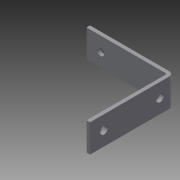
# Autodesk Inventor part: Gusset
Saved by Autodesk Inventor 2013 (Build 170138000, 138)
## iProperties
Created: 2013-01-31
Part Number: Gusset
Material: Generic
Document SubType Name: Sheet Metal
Designer: actoennies
Density: 1 g/cm^3
Flat Pattern Width: 2.54 cm
Flat Pattern Length: 14.7699 cm
Flat Pattern Area: 37.5156 cm^2
Sheet Metal Rule: Default
Sheet Metal Width: 1.000 in
Sheet Metal Length: 5.815 in
Sheet Metal Area: 5.815 in^2
Mass: 11.48 g
Surface Area: 86.0215 cm^2
Volume: 11.48 cm^3
Author: actoennies
Autodesk Inventor part; units mm, degrees
note: some values were not read from the file. Left out: dimensions or parameters whose unit could not be read.
ref_plane "YZ Plane" through (0, 0, 0) normal (1, 0, 0) x (0, 1, 0)
ref_plane "XZ Plane" through (0, 0, 0) normal (0, 1, 0) x (-1, 0, 0)
ref_plane "XY Plane" through (0, 0, 0) normal (0, 0, 1) x (1, 0, 0)
sketch "Sketch1" plane through (0, 0, 0) normal (0, 0, 1) x (1, 0, 0)
  line L0 (0, 0) -> (147.699314, 0)
  line L1 (147.699314, -25.4) -> (0, -25.4)
  line L2 (0, 0) -> (73.8378, 0)
  line L3 (73.8378, 0) -> (73.8378, -3.175)
  line L4 (73.8378, -3.175) -> (72.2503, -3.175)
  line L5 (72.2503, -3.175) -> (72.2503, -9.525)
  line L6 (72.2503, -9.525) -> (75.4253, -9.525)
  line L7 (75.4253, -9.525) -> (75.4253, -3.175)
  line L8 (75.4253, -3.175) -> (73.8378, -3.175)
  line L9 (73.849657, -25.4) -> (73.849657, -22.225)
  line L10 (73.849657, -22.225) -> (72.2503, -22.225)
  line L11 (72.2503, -22.225) -> (72.2503, -15.875)
  line L12 (72.2503, -15.875) -> (75.4253, -15.875)
  line L13 (75.4253, -15.875) -> (75.4253, -22.225)
  line L14 (75.4253, -22.225) -> (73.849657, -22.225)
sketch "Sketch3" plane through (73.025, 0, 76.2) normal (-1, 0, 0) x (0, 0, 1)
  line L0 (0, 0) -> (-71.755, 0) projected
  line L1 (0, 0) -> (0, 25.4) projected
  circle A0 centre (-12.7, 12.7) radius 3.3782
  circle A1 centre (-63.5, 12.7) radius 3.3782
  point P0 (-76.2, 0)
  dimension "d19" = 6.7564
  dimension "d20" = 6.7564
  dimension "d22" = 12.7
  dimension "d23" = 12.7
  dimension "d24" = 12.7
  dimension "d27" = 50.8
  constraints: 2 centre point
  measures "d19" diameter of A0
  measures "d20" diameter of A1
  measures "d22" distance from line of L1 A0.centre
  measures "d23" distance from line of L0 A0.centre
  measures "d24" distance from line of L0 A1.centre
  measures "d27" distance of A0.centre A1.centre
sketch "Sketch1 outline for Plate1" plane through (0, 0, 0) normal (0, 0, 1) x (1, 0, 0)
  line L0 (0, 0) -> (0, 25.4)
  line L1 (76.2, 0) -> (0, 0)
  line L2 (0, 25.4) -> (76.2, 25.4)
  line L3 (76.2, 25.4) -> (76.2, 0)
  circle A0 centre (12.7, 12.7) radius 3.3782
  circle A1 centre (63.5, 12.7) radius 3.3782
extrude "Plate1" add sketch "Sketch1 outline for Plate1" along normal blind 3.175
sketch "Sketch2" plane through (73.025, 25.4, 0) normal (1, 0, 0) x (0, 1, 0)
  line L0 (-25.4, 0) -> (0, 0)
  line L1 (0, 0) -> (0, 76.2)
  line L2 (0, 76.2) -> (-25.4, 76.2)
  line L3 (-25.4, 76.2) -> (-25.4, 0)
  constraints: 6 end point, 1 horizontal, 1 perpendicular, 1 vertical
edge flange "Flange1" height 76.2 angle 90 thickness 3.175 bend radius 1.27 thickness toward (1, 0, 0) relief tear relief width 3.175 relief depth 1.5875 edges at (76.2, 12.7, 3.175) wall of the first edge with corners at (73.025, 0, 0) (73.025, 25.4, 0) (73.025, 25.4, 76.2) (73.025, 0, 76.2)
bend "Bend1"
corner "Corner1"
extrude "Cut1" cut sketch "Sketch3" against normal blind 3.175
equation "\"d9\" = BendReliefWidth"
equation "\"d10\" = BendReliefDepth"
equation "\"d11\" = MinimumRemnant"
equation "\"d12\" = BendRadius"
equation "\"d16\" = CornerReliefSize"
equation "\"d17\" = GapSize"
equation "\"d18\" = JacobiRadiusSize"
equation "\"BendRadius\" = Thickness"
equation "\"BendReliefWidth\" = Thickness"
equation "\"BendReliefDepth\" = 0.5 * Thickness"
equation "\"CornerReliefSize\" = 4 * Thickness"
equation "\"MinimumRemnant\" = 2 * Thickness"
equation "\"TransitionRadius\" = BendRadius"
equation "\"JacobiRadiusSize\" = BendRadius"
equation "\"GapSize\" = Thickness"
equation "\"d8\" = BendRadius"
equation "\"d7\" = Thickness"
equation "\"Thickness\" = 3.175"
body "Solid1"
